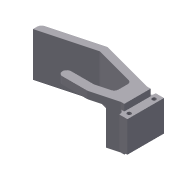
# Autodesk Inventor part: Right Hand
Saved by Autodesk Inventor 2011 (Build 150239000, 239)
## iProperties
Created: 2010-11-26
Part Number: Right Hand
Document SubType Name: Modeling
Designer: Milton
Density: 2.71 g/cm^3
Mass: 54.0022 g
Surface Area: 86.7378 cm^2
Volume: 19.927 cm^3
Material: Aluminum-6061
Author: Milton
Autodesk Inventor part; units mm, degrees
ref_plane "YZ Plane" through (0, 0, 0) normal (1, 0, 0) x (0, 1, 0)
ref_plane "XZ Plane" through (0, 0, 0) normal (0, 1, 0) x (-1, 0, 0)
ref_plane "XY Plane" through (0, 0, 0) normal (0, 0, 1) x (1, 0, 0)
sketch "Sketch1" plane through (0, 0, 0) normal (0, 0, 1) x (1, 0, 0)
  line L0 (52.1089, 41.9337) -> (16.0623, 32.275)
  line L1 (81.0151, 18.2189) -> (81.0151, 29.0119)
  line L2 (81.0151, 29.0119) -> (52.1089, 36.7573)
  line L3 (52.1089, 36.7573) -> (16.0623, 27.0986)
  line L4 (16.0623, 32.275) -> (16.0623, 27.0986)
  line L5 (71.0038, 9.1932) -> (89.0623, 14.032)
  line L6 (71.0038, 9.1932) -> (54.0038, 9.1932)
  line L7 (54.0092, 15.1932) -> (69.7233, 15.1932)
  arc A0 (54.0092, 15.1932) -> (54.0038, 9.1932) centre (54.0065, 12.1932) ccw
  line L8 (69.7233, 15.1932) -> (81.0151, 18.2189)
  line L9 (52.1089, 41.9337) -> (89.0623, 32.032)
  line L10 (97.0623, 35.532) -> (97.0623, 10.532)
  circle A1 centre (94.2623, 31.5608) radius 1.35 projected
  circle A2 centre (94.2623, 14.5608) radius 1.35 projected
  line L11 (89.0623, 32.032) -> (91.4623, 32.032)
  line L12 (91.4623, 32.032) -> (91.4623, 35.532)
  line L13 (91.4623, 35.532) -> (97.0623, 35.532)
  line L14 (89.0623, 14.032) -> (91.4623, 14.032)
  line L15 (91.4623, 14.032) -> (91.4623, 10.532)
  line L16 (91.4623, 10.532) -> (97.0623, 10.532)
  point P0 (0, 0)
  dimension "d0" = 5
  dimension "d1" = 6
  dimension "d2" = 5
  dimension "d3" = 75
  dimension "d4" = 150
  dimension "d5" = 18
  dimension "d6" = 15
  dimension "d28" = 25
  dimension "d30" = 5.6
  dimension "d31" = 5.6
  constraints: 34 end point, 5 parallel, 3 perpendicular, 2 point on circle, 2 vertical, 1 centre point, 1 horizontal
  measures "d0" distance between parallel lines of L0 L3
  measures "d1" distance between parallel lines of L6 L7
  measures "d2" distance between parallel lines of L9 L2
  measures "d3" angle of L1 L2
  measures "d4" angle of L2 L3
  measures "d5" distance of L9.end L5.end
  measures "d6" angle of L6 L5
  measures "d28" distance of L10.start L10.end
  measures "d30" distance of L12.end L10.start
  measures "d31" distance of L15.end L10.end
extrude "Extrusion1" add sketch "Sketch1" along normal blind 30
sketch "Sketch3" plane through (0, 0, 0) normal (0, 0, -1) x (-1, 0, 0)
  line L0 (-81.0151, 18.2189) -> (-46.6558, 18.2189)
  line L1 (-46.6558, 18.2189) -> (-46.6558, 4.635)
  line L2 (-46.6558, 4.635) -> (-81.0151, 4.635)
  line L3 (-81.0151, 4.635) -> (-81.0151, 18.2189)
  point P0 (0, 0)
  constraints: 8 end point, 2 parallel, 1 horizontal, 1 perpendicular
extrude "Extrusion2" cut sketch "Sketch3" against normal blind 25
fillet "Fillet1" radius 3 7 edges at (81.0151, 29.0119, 15) (81.0151, 18.2189, 27.5) (69.7233, 15.1932, 27.5) (52.1089, 36.7573, 15) (52.1089, 41.9337, 15) (16.0623, 32.275, 15) (71.0038, 9.1932, 27.5)
sketch "Sketch6" plane through (91.4623, 35.532, 0) normal (0, 1, 0) x (1, 0, 0)
  line L0 (0, 0) -> (0, -30) projected
  line L1 (5.6, 0) -> (0, 0)
  line L2 (0, 0) -> (0, -4.5)
  line L3 (0, -4.5) -> (5.6, -4.5)
  line L4 (5.6, -4.5) -> (5.6, 0)
  line L5 (5.6, -30) -> (0, -30)
  line L6 (0, -30) -> (0, -25.5)
  line L7 (0, -25.5) -> (5.6, -25.5)
  line L8 (5.6, -25.5) -> (5.6, -30)
  point P0 (-91.4623, 0)
  dimension "d32" = 4.5
  dimension "d33" = 5.6
  dimension "d34" = 4.5
  constraints: 16 end point, 4 parallel, 2 horizontal, 2 perpendicular, 1 point on line
  measures "d32" distance of L2.end L1.end
  measures "d33" distance of L6.end L7.end
  measures "d34" distance of L5.end L6.end
extrude "Extrusion5" cut sketch "Sketch6" against normal through all
fillet "Fillet2" radius 3 2 edges at (91.4623, 32.032, 15) (91.4623, 14.032, 15)
body "Solid1"
